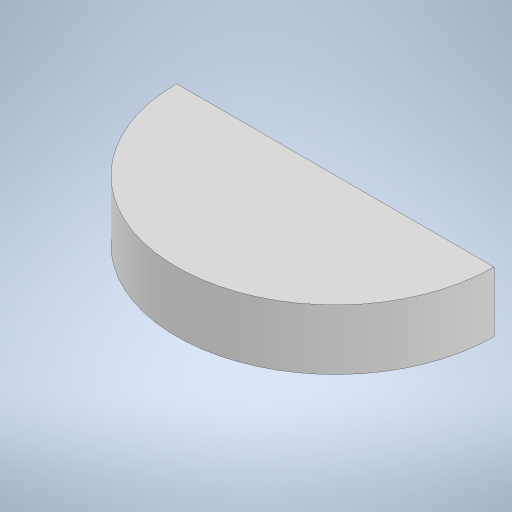
# Autodesk Inventor part: Tapa2
Saved by Autodesk Inventor 2024 (Build 280153000, 153)
## iProperties
Created: 2024-05-21
Part Number: Tapa2
Material: Genérico
Document SubType Name: Modeling
Designer: psepu
Density: 1 g/cm^3
Appearance: Valor por defecto
Author: psepu
Autodesk Inventor part; units mm, degrees
ref_plane "YZ Plane" through (0, 0, 0) normal (1, 0, 0) x (0, 1, 0)
ref_plane "XZ Plane" through (0, 0, 0) normal (0, 1, 0) x (-1, 0, 0)
ref_plane "XY Plane" through (0, 0, 0) normal (0, 0, 1) x (1, 0, 0)
sketch "Boceto1" plane through (0, 0, 0) normal (0, 0, 1) x (1, 0, 0)
  line L0 (0, 35) -> (0, 38)
  line L1 (0, 38) -> (-100, 38)
  line L2 (-100, 38) -> (-100, 0)
  line L3 (-100, 0) -> (-96.8, 0)
  line L4 (-96.8, 0) -> (-96.8, 35)
  line L5 (-96.8, 35) -> (-93.4, 35)
  line L6 (-93.4, 35) -> (-93.4, 0)
  line L7 (-93.4, 0) -> (-90.2, 0)
  line L8 (-90.2, 0) -> (-90.2, 35)
  line L9 (-90.2, 35) -> (0, 35)
  point P0 (0, 0)
  dimension "d0" = 38
  dimension "d1" = 100
  dimension "d2" = 3.2
  dimension "d3" = 35
  dimension "d4" = 3.4
  dimension "d5" = 3.2
  constraints: 20 end point, 6 perpendicular, 4 point on line, 1 horizontal, 1 vertical
  measures "d0" distance of point (0, 0) L0.end
  measures "d1" distance of L0.end L1.end
  measures "d2" distance of L2.end L3.end
  measures "d3" distance of L3.end L4.end
  measures "d4" distance of L4.end L5.end
  measures "d5" distance of L6.end L7.end
revolve "Revolución1" add sketch "Boceto1" angle 180 about axis through (0, 35, 0) along (0, 1, 0)
